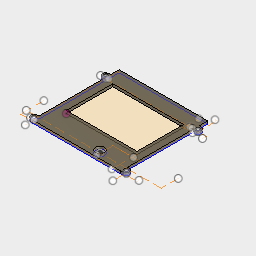
bart pro xl glcd case face (Autodesk Fusion 360 design; units mm, degrees)
Autodesk Fusion 360 part; units mm, degrees
sketch "Sketch1" plane through (0, 0, 0) normal (0, 0, 1) x (1, 0, 0)
  line L0 (0, 0) -> (79, 0)
  line L1 (79, 0) -> (79, 52)
  line L2 (79, 52) -> (0, 52)
  line L3 (0, 52) -> (0, 0)
  line L4 (79, 52) -> (79, 69) construction
  line L5 (89, 69) -> (-10, 69)
  line L6 (79, 52) -> (89, 52) construction
  line L7 (79, 0) -> (79, -28) construction
  line L8 (89, -28) -> (80.3854, -28)
  line L9 (80.3854, -28) -> (-10, -28)
  line L10 (125.2435, -0.1844) -> (125.2435, -19.1844) construction
  line L11 (89, -4.9062) -> (66, -4.9062) construction
  circle A0 centre (57, -19.1844) radius 5
  line L12 (89, 77.1159) -> (91, 77.1159) construction
  line L13 (-10, 69) -> (-12, 69) construction
  line L14 (-12, 69) -> (-12, -33.8581) construction
  line L15 (100.1288, 52.0577) -> (100.1288, 56.0577) construction
  line L16 (100.1288, 56.0577) -> (84.7906, 56.0577) construction
  circle A1 centre (91, 56.0577) radius 2
  line L17 (91, 59.5577) -> (89, 59.5577)
  line L18 (91, 52.5577) -> (89, 52.5577)
  arc A2 (91, 52.5577) -> (91, 59.5577) centre (91, 56.0577) ccw
  line L19 (89, 69) -> (89, 59.5577)
  line L20 (81.9494, 56.0577) -> (-17.7136, 56.0577) construction
  circle A3 centre (-12, 56.0577) radius 2
  line L21 (-12, 59.5577) -> (-10, 59.5577)
  line L22 (-12, 52.5577) -> (-10, 52.5577)
  arc A4 (-12, 59.5577) -> (-12, 52.5577) centre (-12, 56.0577) ccw
  line L23 (-10, 69) -> (-10, 57.5577)
  line L24 (-25.0828, 0.0131) -> (-25.0828, -25.9869) construction
  line L25 (-10, 52.5577) -> (-10, -20.4869)
  line L26 (89, 52.5577) -> (89, -20.4901)
  line L27 (105.1865, -25.9869) -> (105.1865, -23.9869) construction
  line L28 (91, -27.4901) -> (89, -28)
  arc A5 (91, -27.4901) -> (91, -20.4901) centre (91, -23.9901) ccw
  line L29 (-16.0067, -25.9869) -> (-16.0067, -23.9869) construction
  line L30 (-12, -20.4869) -> (-10, -20.4869)
  line L31 (-12, -27.4869) -> (-10, -28)
  arc A6 (-12, -20.4869) -> (-12, -27.4869) centre (-12, -23.9869) ccw
  line L32 (66, -4.9062) -> (57, -4.9062) construction
  line L33 (66, -4.9062) -> (80, -4.9062) construction
  line L34 (57, -4.9062) -> (57, -22.9837) construction
  circle A7 centre (-12, -23.9869) radius 2
  line L35 (91, -20.4901) -> (89, -20.4901)
  line L36 (91, 77.1159) -> (91, 52.5577) construction
  line L37 (91, -25.9869) -> (91, -38.9824) construction
  line L38 (125.2435, -19.1844) -> (91, -19.1844) construction
  line L39 (89, -19.1844) -> (-25.5617, -19.1844) construction
  circle A8 centre (91, -23.9901) radius 2
  line L40 (-25.0828, -25.9869) -> (79, -25.9869) construction
  line L41 (90.8872, -25.9869) -> (91.1128, -25.9869) construction
  line L42 (93.8745, -25.9869) -> (105.1865, -25.9869) construction
  dimension "d1" = 79
  dimension "d2" = 52
  dimension "d3" = 17
  dimension "d4" = 10
  dimension "d6" = 28
  dimension "d7" = 19
  dimension "d8" = 23
  dimension "d9" = 10
  dimension "d11" = 2
  dimension "d12" = 2
  dimension "d13" = 4
  dimension "d14" = 4
  dimension "d15" = 7
  dimension "d16" = 4
  dimension "d17" = 7
  dimension "d24" = 2
  dimension "d26" = 7
  dimension "d27" = 2
  dimension "d29" = 7
  dimension "d30" = 180
  dimension "d31" = 9
  dimension "d32" = 4
  dimension "d34" = 4
  constraint horizontal L0
  constraint vertical L1
  constraint horizontal L2
  constraint vertical L3
  constraint perpendicular L4 L5
  constraint perpendicular L5 L19
  constraint coincident L19
  constraint perpendicular L8 L19
  constraint perpendicular L7 L9
  constraint perpendicular L9 L23
  constraint perpendicular L19 L38
  constraint coincident L38
  constraint perpendicular L12 L36
  constraint perpendicular L13 L14
  constraint perpendicular L16 L19
  constraint coincident L16
  constraint coincident L36
  constraint concentric A1 A2
  constraint tangent L17 A2
  constraint perpendicular L17 L19
  constraint tangent L18 A2
  constraint collinear L19 L26
  constraint perpendicular L4 L20
  constraint coincident L20
  constraint coincident L14
  constraint concentric A3 A4
  constraint coincident L23
  constraint tangent L21 A4
  constraint perpendicular L21 L23
  constraint tangent L22 A4
  constraint collinear L23 L25
  constraint perpendicular L36 L40
  constraint perpendicular L27 L40
  constraint coincident L40
  constraint perpendicular L29 L40
  constraint tangent L30 A6
  constraint horizontal L33
  constraint perpendicular L34 L38
  constraint coincident L34
  constraint concentric A6 A7
  constraint tangent A5 L35
  constraint perpendicular L26 L35
  constraint collinear L36 L37
  constraint coincident L26
  constraint collinear L38 L39
  constraint concentric A5 A8
  constraint coincident L7
  constraint coincident A8
  constraint collinear L40 L41
  constraint coincident A5
  constraint collinear L41 L42
  measures "d9" diameter of A0
  measures "d14" diameter of A1
  measures "d15" diameter of A2
  measures "d16" diameter of A3
  measures "d17" diameter of A4
  measures "d26" diameter of A5
  measures "d29" diameter of A6
  measures "d30" angle of L32 L33
  measures "d32" diameter of A7
  measures "d34" diameter of A8
extrude "Extrude4" add sketch "Sketch1" along normal blind 3
